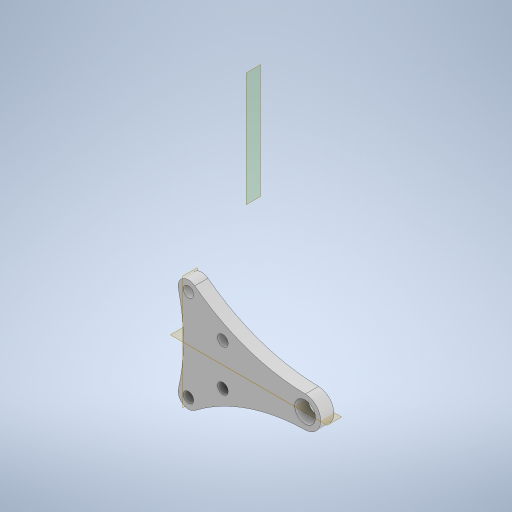
# Autodesk Inventor part: XZ Plate2
Saved by Autodesk Inventor 2023.1 (Build 271208000, 208)
## iProperties
Created: 2022-10-29
Part Number: XZ Plate2
Material: Generic
Document SubType Name: Modeling
Designer: nicol
Density: 1 g/cm^3
Appearance: Default
Author: nicol
Autodesk Inventor part; units mm, degrees
ref_plane "XY Plane" through (0, 0, 0) normal (0, 0, 1) x (1, 0, 0)
sketch "Sketch1" plane through (0, 0, 0) normal (0, 0, 1) x (1, 0, 0)
  line L0 (-20, 150) -> (20, 150) construction
  line L1 (20, 150) -> (20, -150) construction
  line L2 (20, -150) -> (-20, -150) construction
  line L3 (-20, -150) -> (-20, 150) construction
  circle A0 centre (-28.08, 22) radius 10.72 construction
  circle A1 centre (-28.08, -22) radius 10.72 construction
  circle A2 centre (28.08, 0) radius 10.72 construction
  line L4 (38.8, 14.9853) -> (38.8, -13.1126) construction
  circle A3 centre (28.08, 0) radius 7.5
  circle A4 centre (-28.08, 22) radius 5
  circle A5 centre (-28.08, -22) radius 5
  arc A6 (-32.9441, -20.8421) -> (-32.9441, 20.8421) centre (-120.4975, 0) ccw
  arc A7 (-25.0444, 25.9731) -> (28.1966, 7.4991) centre (29.5961, 97.4882) ccw
  arc A8 (28.1966, -7.4991) -> (-25.0444, -25.9731) centre (29.5961, -97.4882) ccw
  line L5 (-30.4975, 3.8118) -> (-30.4975, -3.8118) construction
  line L6 (0, 150) -> (0, -150) construction
  line L7 (-62, -108) -> (-20, -108) construction
  line L8 (-20, -108) -> (-20, -150) construction
  line L9 (-20, -150) -> (-62, -150) construction
  line L10 (-62, -150) -> (-62, -108) construction
  line L11 (-62, 150) -> (-20, 150) construction
  line L12 (-20, 150) -> (-20, 108) construction
  line L13 (-20, 108) -> (-62, 108) construction
  line L14 (-62, 108) -> (-62, 150) construction
  circle A9 centre (-41, -129) radius 6 construction
  line L15 (-70.4975, 7.5) -> (-30.4975, 7.5)
  line L16 (-30.4975, 7.5) -> (-30.4975, -7.5)
  line L17 (-30.4975, -7.5) -> (-70.4975, -7.5)
  line L18 (-70.4975, -7.5) -> (-70.4975, 7.5)
  point P0 (0, 0)
  point P1 (20, 0)
  point P2 (-29.8, 0)
  point P3 (-20, 0)
  point P4 (-62, -129)
  point P5 (-41, -108)
  point P6 (-30.4975, 0)
  point P7 (-62.9975, 0)
  point P8 (-37.9975, 0)
  point P9 (-70.4975, 0)
  point P10 (-30.8106, -7.5)
  point P11 (-30.8106, 7.5)
  point P12 (-11.5, 10)
  point P13 (-11.5, -10)
  dimension "d0" = 40
  dimension "d1" = 300
  dimension "d2" = 21.44
  dimension "d3" = 22
  dimension "d4" = 22
  dimension "d5" = 58.8
  dimension "d6" = 28.08
  dimension "d7" = 28.08
  dimension "d9" = 90
  dimension "d12" = 15
  dimension "d38" = 10
  dimension "d40" = 42
  dimension "d41" = 12
  dimension "d42" = 15
  dimension "d43" = 40
  dimension "d44" = 25
  dimension "d45" = 7.5
  dimension "d46" = 7.5
  dimension "d48" = 90
  dimension "d49" = 16.58
  dimension "d50" = 12
  dimension "d51" = 10
  constraints: 38 end point, 12 point on circle, 10 centre point, 9 midpoint, 9 tangent, 8 parallel, 7 horizontal alignment, 4 collinear, 4 equal radius, 4 horizontal, 4 perpendicular, 4 vertical alignment, 3 equal length, 2 vertical
  measures "d0" distance of L0.start L0.end
  measures "d1" distance of L0.end L1.end
  measures "d2" diameter of A2
  measures "d3" vertical distance of point (0, 0) A1.centre
  measures "d4" vertical distance of A0.centre point (0, 0)
  measures "d5" distance between parallel lines of L3 L4
  measures "d6" distance of A2.centre point (0, 0)
  measures "d7" horizontal distance of point (0, 0) A0.centre
  measures "d9" radius of A7
  measures "d12" diameter of A3
  measures "d38" diameter of A4
  measures "d40" distance of L11.start L11.end
  measures "d41" diameter of A9
  measures "d42" distance of L17.end L15.start
  measures "d43" distance of L15.start L15.end
  measures "d44" distance of point (-37.998, 0) point (-62.998, 0)
  measures "d45" distance from line of L5 point (-37.998, 0)
  measures "d46" distance from line of L18 point (-62.998, 0)
  measures "d48" radius of A6
  measures "d49" horizontal distance of point (-11.5, 10) A0.centre
  measures "d50" vertical distance of A0.centre point (-11.5, 10)
  measures "d51" vertical distance of point (-11.5, -10) point (-20, 0)
extrude "Extrusion1" add sketch "Sketch1" against normal blind 6.35 contours A3 | A3 A8 A5 A6 L17 L16 L15 A4 A7 | A4 | A5 | L15 L16 A6 | A6 L16 L17
hole "Hole1" at (-28.08, 22, 0) at (-28.08, -22, 0) direction (0, 0, -1) diameter 5 end through all
hole "Hole3" at (28.08, 0, 0) direction (0, 0, -1) diameter 10 end through all
ref_plane "Work Plane2" through (-30.4975, 0, 0) normal (1, 0, 0) x (0, 1, 0)
ref_plane "Work Plane3" through (0, 150, 0) normal (-1, 0, 0) x (0, -1, 0)
hole "Hole4" at (-62.9975, 0, 0) at (-37.9975, 0, 0) at (-11.5, 10, 0) at (-11.5, -10, 0) direction (0, 0, -1) diameter 5.1 end through all
equation "\"d4\" = d3"
equation "\"d7\" = d6"
equation "\"d46\" = d45"
body "Solid1"
